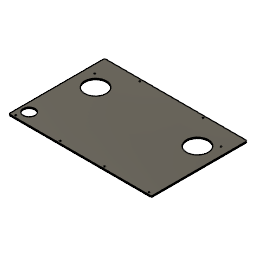
RAMSidePlate (Autodesk Fusion 360 design; units mm, degrees)
part number: 2026-09-01-00-57-05-691
part number: 2026-09-01-00-57-06-495
Autodesk Fusion 360 part; units mm, degrees
sketch "Cut_Profile_1to1_QTY1" plane through (0, 0, 0) normal (0, 0, 1) x (1, 0, 0) in component "RAMSidePlate"
  line L0 (-178.5, -122) -> (178.5, -122)
  arc A0 (178.5, -122) -> (181.5, -119) centre (178.5, -119) ccw
  line L1 (181.5, -119) -> (181.5, 119)
  arc A1 (181.5, 119) -> (178.5, 122) centre (178.5, 119) ccw
  line L2 (178.5, 122) -> (-178.5, 122)
  arc A2 (-178.5, 122) -> (-181.5, 119) centre (-178.5, 119) ccw
  line L3 (-181.5, 119) -> (-181.5, -119)
  arc A3 (-181.5, -119) -> (-178.5, -122) centre (-178.5, -119) ccw
  circle A4 centre (-129.5, 47) radius 27.5
  circle A5 centre (129.5, 47) radius 27.5
  circle A6 centre (-159.5, -92) radius 15
  circle A7 centre (-86.5, 116) radius 1.6
  circle A8 centre (74.5, 116) radius 1.6
  circle A9 centre (-160.5, 76) radius 1.6
  circle A10 centre (160.5, 76) radius 1.6
  circle A11 centre (-169.5, -116) radius 1.6
  circle A12 centre (-56.5, -116) radius 1.6
  circle A13 centre (56.5, -116) radius 1.6
  circle A14 centre (169.5, -116) radius 1.6
extrude "Acrylic_Plate_3mm" add sketch "Cut_Profile_1to1_QTY1" along normal blind 3 in component "RAMSidePlate"
component "RAMSidePlate" placed x (1, 0, 0) y (0, 1, 0) z (0, 0, 1) at (0, 0, 0)
equation "mainboardLength = 355.0 mm" comment "Motherboard envelope length"
equation "mainboardWidth = 236.0 mm" comment "Motherboard envelope width"
equation "acrylicThickness = 3.0 mm" comment "Acrylic sheet thickness"
equation "assemblyClearance = 1.0 mm" comment "Clearance between motherboard and side wall"
equation "sideWallThickness = 3.0 mm" comment "Reserved side-wall thickness"
equation "plateLength = mainboardLength + 2 * ( assemblyClearance + sideWallThickness )" comment "Finished plate length"
equation "plateWidth = mainboardWidth + 2 * ( assemblyClearance + sideWallThickness )" comment "Finished plate width"
equation "cornerRadius = 3.0 mm" comment "Portable-safe outside corner radius"
equation "ventDiameter = 55.0 mm" comment "Diameter of each fully open fan cutout"
equation "ventOffsetTopFromBoard = 71.0 mm" comment "Vent center offset from motherboard top edge"
equation "ventOffsetSideFromBoard = 48.0 mm" comment "Vent center offset from motherboard left/right edge"
equation "ventCenterOffsetX = plateLength / 2 - ( ventOffsetSideFromBoard + assemblyClearance + sideWallThickness )" comment "Absolute X offset of either vent center"
equation "ventCenterOffsetY = plateWidth / 2 - ( ventOffsetTopFromBoard + assemblyClearance + sideWallThickness )" comment "Y offset of both vent centers"
equation "mountHoleDiameter = 3.2 mm" comment "M3 screw clearance-hole diameter"
equation "accessHoleDiameter = 30.0 mm" comment "Diameter of the lower-left access opening"
equation "accessHoleOffsetLeft = 22.0 mm" comment "Access-opening center from the left plate edge"
equation "accessHoleOffsetBottom = 30.0 mm" comment "Access-opening center from the bottom plate edge"
equation "topMountOffsetSide = 21.0 mm" comment "Top mount centers from left/right plate edges"
equation "topMountOffsetTop = 46.0 mm" comment "Top mount centers from top plate edge"
equation "newTopHoleOffsetTop = 6.0 mm" comment "New M3 hole centers from top plate edge"
equation "newTopHole1OffsetLeft = 95.0 mm" comment "New left M3 hole center from left plate edge"
equation "newTopHole2OffsetRight = 107.0 mm" comment "New right M3 hole center from right plate edge"
equation "bottomMountOffsetLeft = 12.0 mm" comment "Leftmost bottom mount center from the left plate edge"
equation "bottomMountOffsetRight = 12.0 mm" comment "Rightmost bottom mount center from the right plate edge"
equation "bottomMountOffsetBottom = 6.0 mm" comment "Four bottom mount centers from bottom plate edge"
equation "bottomMountSpacing = ( plateLength - bottomMountOffsetLeft - bottomMountOffsetRight ) / 3" comment "Equal spacing between the four bottom mounts"
equation "cutQuantity = 1" comment "Cut one RAM-side plate"
equation "d28 = acrylicThickness"
named bodies: "RAMSidePlate_QTY1"
